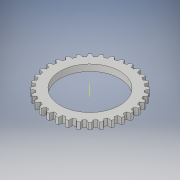
# Autodesk Inventor part: tableGear
Saved by Autodesk Inventor 2018 (Build 220112000, 112)
## iProperties
Created: 2018-04-17
Part Number: tableGear
Material: Generic
Document SubType Name: Modeling
Designer: Cole Tucker
Density: 1 g/cm^3
Appearance: Default
Author: Cole Tucker
Autodesk Inventor part; units mm, degrees
ref_plane "YZ Plane" through (0, 0, 0) normal (1, 0, 0) x (0, 1, 0)
ref_plane "XZ Plane" through (0, 0, 0) normal (0, 1, 0) x (-1, 0, 0)
ref_plane "XY Plane" through (0, 0, 0) normal (0, 0, 1) x (1, 0, 0)
sketch "Sketch1" plane through (0, 0, 0) normal (0, 1, 0) x (-1, 0, 0)
  circle A0 centre (0, 0) radius 29.21
  circle A1 centre (0, 0) radius 38.1
  dimension "d0" = 58.42
  dimension "d1" = 76.2
  constraints: 2 centre point, 2 coincident
  measures "d0" diameter of A0
  measures "d1" diameter of A1
extrude "Extrusion1" add sketch "Sketch1" along normal blind 6.35
sketch "Sketch2" plane through (0, 6.35, 0) normal (0, 1, 0) x (1, 0, 0)
  circle A0 centre (0, 0) radius 29.21 projected
  circle A1 centre (0, 0) radius 38.1 projected
  circle A2 centre (0, 0) radius 38.1 projected
  line L0 (-38.1, 0) -> (-41.275, 0)
  line L1 (-41.275, 0) -> (-41.275, 1.27)
  line L2 (-38.1, 0) -> (-37.3971, 0)
  line L3 (-37.3971, 0) -> (-37.3971, 2.54)
  line L4 (-37.3971, 2.54) -> (-41.275, 1.27)
  line L5 (-37.3971, 0) -> (-37.3971, -2.54)
  line L6 (-41.275, 0) -> (-41.275, -1.27)
  line L7 (-41.275, -1.27) -> (-37.3971, -2.54)
  dimension "d4" = 3.175
  dimension "d5" = 1.27
  dimension "d6" = 2.54
  dimension "d7" = 2.54
  dimension "d8" = 1.27
  constraints: 16 end point, 2 horizontal, 2 perpendicular, 1 horizontal alignment, 1 point on line, 1 vertical, 1 other
  measures "d4" distance of L0.start L0.end
  measures "d5" distance of L0.end L1.end
  measures "d6" distance of L2.end L3.end
  measures "d7" distance of L2.end L5.end
  measures "d8" distance of L0.end L6.end
extrude "Extrusion2" add sketch "Sketch2" against normal blind 6.35 contours L4 L3 L2 A1 | A1 L0 L1 L4 | L7 L6 L0 A1 | A1 L2 L5 L7
pattern_circular "Circular Pattern1" count 32 over 360 about axis through (0, 0, 0) along (0, 1, 0) of "Extrusion2"
body "Solid1"
